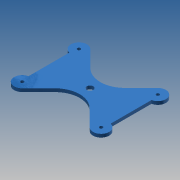
# Autodesk Inventor part: Protector
Saved by Autodesk Inventor 2017 (Build 210142000, 142)
## iProperties
Part Number: Protector
Material: Genérico
Document SubType Name: Modeling
Designer: Leo
Density: 1 g/cm^3
Appearance: Cian
Description: Aluminio compuesto routeado CNC
Author: Leo
Autodesk Inventor part; units mm, degrees
ref_plane "YZ Plane" through (0, 0, 0) normal (1, 0, 0) x (0, 1, 0)
ref_plane "XZ Plane" through (0, 0, 0) normal (0, 1, 0) x (-1, 0, 0)
ref_plane "XY Plane" through (0, 0, 0) normal (0, 0, 1) x (1, 0, 0)
sketch "Boceto1" plane through (0, 0, 0) normal (0, 0, 1) x (1, 0, 0)
  circle A0 centre (23.266, -35) radius 2 projected
  circle A1 centre (120.734, -35) radius 2 projected
  circle A2 centre (120.734, 35) radius 2 projected
  line L0 (93.2132, 21.6214) -> (113.6629, 42.0711)
  arc A3 (122.734, 25.202) -> (113.6629, 42.0711) centre (120.734, 35) ccw
  line L1 (122.734, 25.202) -> (122.734, -25.202)
  arc A4 (113.6629, -42.0711) -> (122.734, -25.202) centre (120.734, -35) ccw
  line L2 (113.6629, -42.0711) -> (93.2132, -21.6214)
  line L3 (50.7868, -21.6214) -> (30.3371, -42.0711)
  arc A5 (21.266, -25.202) -> (30.3371, -42.0711) centre (23.266, -35) ccw
  circle A6 centre (72, 0) radius 4 projected
  arc A7 (93.2132, -21.6214) -> (50.7868, -21.6214) centre (72, -42.8346) ccw
  circle A8 centre (23.266, 35) radius 2
  arc A9 (50.7868, 21.6214) -> (93.2132, 21.6214) centre (72, 42.8346) ccw
  line L4 (50.7868, 21.6214) -> (30.3371, 42.0711)
  arc A10 (30.3371, 42.0711) -> (21.266, 25.202) centre (23.266, 35) ccw
  line L5 (21.266, 25.202) -> (21.266, -25.202)
  point P0 (0, 0)
  point P1 (72, -0.4082)
  dimension "d0" = 10
  dimension "d1" = 8
  dimension "d4" = 10
  dimension "d5" = 30
  dimension "d6" = 8
  dimension "d7" = 90
  constraints: 12 end point, 12 point on circle, 8 tangent, 7 centre point, 4 concentric, 4 equal radius, 3 perpendicular, 2 point on line, 2 vertical, 1 horizontal alignment, 1 vertical alignment
  measures "d0" radius of A3
  measures "d1" distance edge to line of A3 L1
  measures "d4" radius of A5
  measures "d5" radius of A7
  measures "d6" distance edge to line of A10 L5
  measures "d7" angle of L3 L2
extrude "Extrusión1" add sketch "Boceto1" along normal blind 4
equation "\"d4\" = d0"
equation "\"d6\" = d1"
